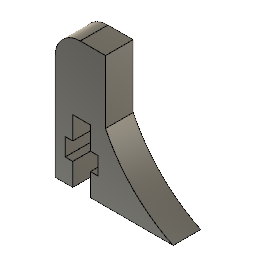
stator_stand v4 (Autodesk Fusion 360 design; units mm, degrees)
Autodesk Fusion 360 part; units mm, degrees
note: some values were not read from the file. Set by a fixed rule: which sketch regions a step uses.
sketch "Sketch1" plane through (0, 0, 0) normal (0, 1, 0) x (1, 0, 0)
  circle A0 centre (0, 0) radius 57.5
  line L0 (-25, -51.7808) -> (25, -51.7808)
  line L1 (51.7808, -25) -> (51.7808, 25)
  line L2 (25, 51.7808) -> (-25, 51.7808)
  line L3 (-51.7808, 25) -> (-51.7808, -25)
  line L4 (-51.7808, 0) -> (-61.7808, 0)
  line L5 (-71.7808, 10) -> (-71.7808, 51.7808)
  line L6 (-71.7808, 51.7808) -> (-25, 51.7808)
  arc A1 (-71.7808, 10) -> (-61.7808, 0) centre (-61.7808, 10) ccw
  line L7 (0, 0) -> (0, 51.7808)
  line L8 (-64.7808, 26.7808) -> (-57.7808, 26.7808)
  line L9 (-57.7808, 26.7808) -> (-57.7808, 51.7808)
  line L10 (-57.7808, 51.7808) -> (-64.7808, 51.7808)
  line L11 (-64.7808, 51.7808) -> (-64.7808, 26.7808)
  line L12 (-67.7808, 35.7808) -> (-54.7808, 35.7808)
  line L13 (-54.7808, 35.7808) -> (-54.7808, 42.7808)
  line L14 (-54.7808, 42.7808) -> (-67.7808, 42.7808)
  line L15 (-67.7808, 42.7808) -> (-67.7808, 35.7808)
  line L16 (-61.2808, 35.7808) -> (-61.2808, 26.7808)
  line L17 (-67.7808, 39.2808) -> (-64.7808, 39.2808)
  line L18 (64.7808, 26.7808) -> (57.7808, 26.7808)
  line L19 (57.7808, 26.7808) -> (57.7808, 51.7808)
  line L20 (64.7808, 51.7808) -> (64.7808, 26.7808)
  line L21 (67.7808, 35.7808) -> (54.7808, 35.7808)
  line L22 (54.7808, 35.7808) -> (54.7808, 42.7808)
  line L23 (67.7808, 42.7808) -> (67.7808, 35.7808)
  line L24 (54.7808, 42.7808) -> (67.7808, 42.7808)
  line L25 (51.7808, 0) -> (61.7808, 0)
  arc A2 (61.7808, 0) -> (71.7808, 10) centre (61.7808, 10) ccw
  line L26 (71.7808, 10) -> (71.7808, 51.7808)
  line L27 (71.7808, 51.7808) -> (25, 51.7808)
  point P0 (-71.7808, 0)
  dimension "d1" = 115
  dimension "d2" = 50
  dimension "d4" = 360
  dimension "d5" = 20
  dimension "d6" = 10
  dimension "d7" = 25
  dimension "d8" = 7
  dimension "d9" = 7
  dimension "d10" = 7
  dimension "d11" = 13
  dimension "d12" = 90
  dimension "d13" = 90
  dimension "d16" = 51.7808
  constraint coincident A0.centre L7.start
  constraint coincident A0 L0.start
  constraint coincident A0 L0.end
  constraint horizontal L0
  constraint midpoint L3 L4.start
  constraint perpendicular L3 L4
  constraint perpendicular L2 L5
  constraint perpendicular L5 L6
  constraint coincident P0 L4
  constraint coincident P0 L5
  constraint tangent L4 A1
  constraint tangent L5 A1
  constraint midpoint L2 L7.end
  constraint horizontal L8
  constraint vertical L9
  constraint horizontal L10
  constraint vertical L11
  constraint coincident L6 L9.end
  constraint horizontal L12
  constraint vertical L13
  constraint horizontal L14
  constraint vertical L15
  constraint midpoint L12 L16.start
  constraint midpoint L8 L16.end
  constraint midpoint L15 L17.start
  constraint midpoint L11 L17.end
  constraint symmetric L2.end L7 L2.start
  constraint symmetric L4.start L7 L25.start
  constraint symmetric L5.end L7 L26.end
  constraint symmetric L4.end L7 L25.end
  constraint symmetric L5.start L7 A2.end
  constraint symmetric A1 L7 A2
  constraint symmetric L7 L8.start L18.start
  constraint symmetric L7 L8.end L18.end
  constraint symmetric L7 L9.end L19.end
  constraint symmetric L7 L10.end L20.start
  constraint symmetric L7 L12.start L21.start
  constraint symmetric L7 L12.end L21.end
  constraint symmetric L7 L13.end L22.end
  constraint symmetric L7 L14.end L23.start
  measures "d1" diameter of A0
  measures "d2" distance of L0.start L0.end
  measures "d5" distance of L4.start P0
  measures "d6" radius of A1
  measures "d7" distance of L8.start L10.end
  measures "d8" distance of L8.start L8.end
  measures "d9" distance of L5 L11
  measures "d10" distance of L12.end L13.end
  measures "d11" distance of L12.start L12.end
  measures "d12" angle of L12 L16
  measures "d13" angle of L15 L17
  measures "d16" distance of A0.centre L7.end
extrude "Extrude1" add sketch "Sketch1" along normal blind 10 contours A0 L1 L25 | A0 L18 L19 L20 L21 L22 L23 L24 L25 A2 L26 L27 | A0 L4 L5 L6 A1 L8 L9 L11 L12 L13 L14 L15 | A0 L3 L4 picked at (55.3786, 2.8629) picked at (-55.3786, 2.8629) makes body 1 at (-63.7808, 0, -12.2603) makes body 2 at (63.7808, 0, -12.2603)
extrude "Extrude2" cut 1 faces at (63.7808, 0, -12.2603) along direction (0, 1, 0) blind 20 on bodies 2 bodies 2
extrude "Extrude3" add 1 faces at (-63.7808, 0, -12.2603) along direction (0, -1, 0) blind 1 on bodies 1 bodies 1 2
